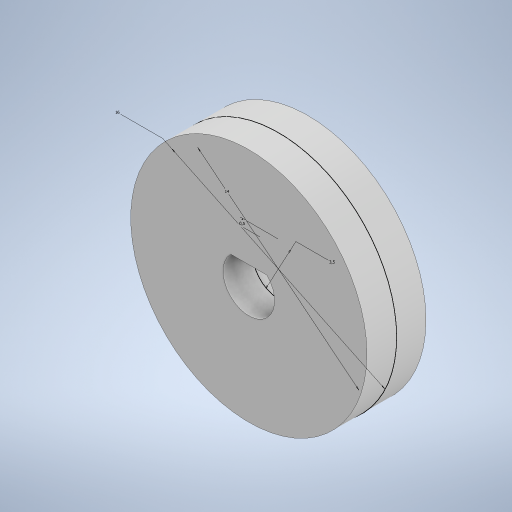
# Autodesk Inventor part: Hudson 1-62C
Saved by Autodesk Inventor 2024.2 (Build 282272000, 272)
## iProperties
Created: 2024-10-07
Part Number: Hudson 1-62C
Material: Genérico
Document SubType Name: Modeling
Designer: Monica Mora
Density: 1 g/cm^3
Appearance: Valor por defecto
Author: Monica Mora
Autodesk Inventor part; units mm, degrees
ref_plane "YZ Plane" through (0, 0, 0) normal (1, 0, 0) x (0, 1, 0)
ref_plane "XZ Plane" through (0, 0, 0) normal (0, 1, 0) x (-1, 0, 0)
ref_plane "XY Plane" through (0, 0, 0) normal (0, 0, 1) x (1, 0, 0)
sketch "Boceto1" plane through (0, 0, 0) normal (0, 0, 1) x (1, 0, 0)
  circle A0 centre (0, 0) radius 8
  circle A1 centre (0, 0) radius 7
  circle A2 centre (0, 0) radius 1.75
  line L0 (-1.2247, 1.25) -> (1.2247, 1.25)
  dimension "d0" = 3.5
  dimension "d1" = 14
  dimension "d2" = 16
  dimension "d3" = 0.5
  constraints: 3 centre point, 3 coincident, 2 end point, 2 point on circle, 1 horizontal
  measures "d0" diameter of A2
  measures "d1" diameter of A1
  measures "d2" diameter of A0
  measures "d3" distance edge to line of A2 L0
extrude "Extrusión1" add sketch "Boceto1" along normal mid plane 4 contours A1 | L0 A2 picked at (0.0645, 1.4131)
extrude "Extrusión2" add sketch "Boceto1" along normal mid plane 4 contours A0
